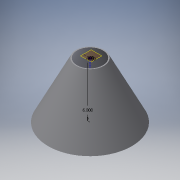
# Autodesk Inventor part: Funnel1
Saved by Autodesk Inventor 2019 (Build 230136000, 136)
## iProperties
Created: 2019-11-21
Part Number: Funnel1
Material: Generic
Document SubType Name: Modeling
Designer: Administrator
Density: 1 g/cm^3
Appearance: Default
Author: Administrator
Autodesk Inventor part; units mm, degrees
ref_plane "YZ Plane" through (0, 0, 0) normal (1, 0, 0) x (0, 1, 0)
ref_plane "XZ Plane" through (0, 0, 0) normal (0, 1, 0) x (-1, 0, 0)
ref_plane "XY Plane" through (0, 0, 0) normal (0, 0, 1) x (1, 0, 0)
sketch "Sketch1" plane through (0, 0, 0) normal (0, 1, 0) x (-1, 0, 0)
  circle A0 centre (0, 0) radius 114.3
  line L0 (0, 0) -> (-114.3, 0)
  dimension "d20" = 228.6
  constraints: 2 end point, 1 coincident, 1 horizontal, 1 horizontal alignment, 2 other
sketch3d "3D Sketch3"
ref_plane "Work Plane6" through (0, 152.4, 0) normal (0, 1, 0) x (0, 0, 1)
sketch "Sketch8" plane through (0, 152.4, 0) normal (0, 1, 0) x (0, 0, 1)
  circle A0 centre (0, 0) radius 38.1
  point P0 (0, 0)
  dimension "d14" = 76.2
  constraints: 1 centre point, 1 coincident
  measures "d14" diameter of A0
loft "Loft1" add profiles "Sketch1", "Sketch8"
shell "Shell1" thickness 2.54 removed faces 2 at (4.3637, 152.4, 0.9393) at (-34.4881, 0, 8.72)
body "Solid2"
